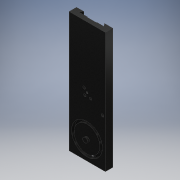
# Autodesk Inventor part: slide ontop of saddle
Saved by Autodesk Inventor 2018 (Build 220112000, 112)
## iProperties
Created: 2017-05-09
Part Number: slide ontop of saddle
Material: Steel, Cast
Document SubType Name: Modeling
Designer: m227586
Density: 7.85 g/cm^3
Appearance: Black Cast
Author: m227586
Autodesk Inventor part; units mm, degrees
ref_plane "YZ Plane" through (0, 0, 0) normal (1, 0, 0) x (0, 1, 0)
ref_plane "XZ Plane" through (0, 0, 0) normal (0, 1, 0) x (-1, 0, 0)
ref_plane "XY Plane" through (0, 0, 0) normal (0, 0, 1) x (1, 0, 0)
sketch "Sketch1" plane through (0, 0, 0) normal (0, 0, 1) x (1, 0, 0)
  line L0 (-7.7614, 0) -> (138.2386, 0)
  line L1 (138.2386, 0) -> (138.2386, 29.6)
  line L2 (-7.7614, 29.6) -> (-7.7614, 0)
  line L3 (-7.7614, 29.6) -> (22.1386, 29.6)
  line L4 (12.489, 18.1) -> (114.8883, 18.1)
  line L5 (22.1386, 29.6) -> (12.489, 18.1)
  line L6 (22.1386, 29.6) -> (41.4586, 29.6) construction
  line L7 (138.2386, 29.6) -> (105.2386, 29.6)
  line L8 (105.2386, 29.6) -> (114.8883, 18.1)
  point P0 (0, 0)
  dimension "d0" = 146
  dimension "d1" = 29.6
  dimension "d2" = 29.9
  dimension "d4" = 130
  dimension "d5" = 33
  dimension "d6" = 50
  constraints: 18 end point, 4 horizontal, 2 perpendicular
  measures "d0" distance of L0.start L0.end
  measures "d1" distance of L0.end L1.end
  measures "d2" distance of L2.start L3.end
  measures "d4" angle of L5 L6
  measures "d5" distance of L1.end L7.end
  measures "d6" angle of L8 L7
extrude "Extrusion1" add sketch "Sketch1" against normal blind 486
sketch "Sketch2" plane through (-7.7614, 29.6, 0) normal (0, 1, 0) x (1, 0, 0)
  line L0 (113, 0) -> (122.6496, 0) projected
  line L1 (124, 486) -> (113, 0)
  line L2 (113, 0) -> (113, 486) projected
  line L3 (113, 486) -> (124, 486)
  line L4 (122.6496, 0) -> (122.6496, 486) projected
  line L5 (113, 486) -> (113, 0)
  line L6 (146, 0) -> (146, 486) projected
  point P0 (7.7614, 0)
  dimension "d9" = 22
  constraints: 6 end point, 1 parallel, 1 perpendicular
  measures "d9" distance of L6.end L1.start
sketch "Sketch3" plane through (-7.7614, 0, 0) normal (0, -1, 0) x (1, 0, 0)
  line L0 (20.2504, -486) -> (122.6496, -486) projected
  line L1 (0, 0) -> (146, 0) projected
  circle A0 centre (71.6943, -409.4001) radius 62.1
  line L2 (71.45, -486) -> (71.4962, -471.5001)
  circle A1 centre (71.6943, -409.4001) radius 52
  circle A2 centre (71.6943, -409.4001) radius 9.51
  circle A3 centre (72.1613, -247.2004) radius 4.1
  point P0 (7.7614, 0)
  dimension "d10" = 124.2
  dimension "d11" = 14.5
  dimension "d12" = 62.1
  dimension "d13" = 104
  dimension "d14" = 19.02
  dimension "d15" = 8.2
  constraints: 4 centre point, 2 coincident, 2 end point, 1 midpoint
  measures "d10" diameter of A0
  measures "d11" distance of L2.start L2.end
  measures "d12" vertical distance of A0.centre L2.end
  measures "d13" diameter of A1
  measures "d14" diameter of A2
  measures "d15" diameter of A3
extrude "Extrusion2" cut sketch "Sketch3" against normal blind 13 contours A0
extrude "Extrusion3" add sketch "Sketch3" along normal blind 7.5 contours A2
extrude "Extrusion4" cut sketch "Sketch3" against normal through all contours A3
sketch "Sketch4" plane through (12.489, 18.1, 0) normal (0, 1, 0) x (1, 0, 0)
  circle A0 centre (51.911, 247.2004) radius 4.1 projected
  circle A1 centre (51.911, 247.2004) radius 9.5
  line L0 (0, 486) -> (102.3993, 486) projected
  line L1 (51.1996, 486) -> (51.1996, 476.6)
  arc A2 (46.6496, 476.6) -> (46.6496, 457.9) centre (46.6496, 467.25) ccw
  arc A3 (55.7496, 457.9) -> (55.7496, 476.6) centre (55.7496, 467.25) ccw
  line L2 (46.6496, 476.6) -> (55.7496, 476.6)
  line L3 (46.6496, 457.9) -> (55.7496, 457.9)
  circle A4 centre (51.1996, 411.4) radius 8.5
  point P0 (-12.489, 0)
  point P1 (51.1996, 476.6)
  dimension "d23" = 19
  dimension "d26" = 9.4
  dimension "d29" = 0
  dimension "d30" = 18.7
  dimension "d31" = 18.7
  dimension "d38" = 17
  dimension "d39" = 46.5
  constraints: 6 end point, 4 centre point, 4 point on circle, 2 coincident, 1 horizontal, 1 midpoint, 1 parallel, 1 vertical
  measures "d23" diameter of A1
  measures "d26" distance of L1.start L1.end
  measures "d29" distance from line of point (51.2, 476.6) L1
  measures "d30" diameter of A2
  measures "d31" diameter of A3
  measures "d38" diameter of A4
  measures "d39" distance from line of A4.centre L3
extrude "Extrusion5" cut sketch "Sketch4" against normal blind 3.7 contours A1
extrude "Extrusion7" cut sketch "Sketch4" against normal blind 6 contours L2 A3 L3 A2
extrude "Extrusion8" cut sketch "Sketch4" against normal blind 3 contours A4
sketch "Sketch5" plane through (-7.7614, 0, 0) normal (0, -1, 0) x (1, 0, 0)
  point P0 (7.7614, 0)
sketch "Sketch6" plane through (-7.7614, 0, 0) normal (0, -1, 0) x (1, 0, 0)
  circle A0 centre (86, -261) radius 5
  line L0 (146, -486) -> (0, -486) projected
  line L1 (146, 0) -> (146, -486) projected
  circle A1 centre (60.5, -235.5) radius 5.5
  line L2 (0, 0) -> (0, -486) projected
  circle A2 centre (134.5, -295.5) radius 5.5
  point P0 (7.7614, 0)
  dimension "d42" = 10
  dimension "d43" = 225
  dimension "d44" = 60
  dimension "d45" = 11
  dimension "d46" = 60.5
  dimension "d47" = 250.5
  dimension "d48" = 11
  dimension "d49" = 190.5
  dimension "d50" = 11.5
  constraints: 3 centre point, 3 coincident
  measures "d42" diameter of A0
  measures "d43" distance from line of L0 A0.centre
  measures "d44" distance from line of L1 A0.centre
  measures "d45" diameter of A1
  measures "d46" distance from line of L2 A1.centre
  measures "d47" distance from line of L0 A1.centre
  measures "d48" diameter of A2
  measures "d49" distance from line of L0 A2.centre
  measures "d50" distance from line of L1 A2.centre
hole "Hole1" at (126.7386, 0, -295.5) direction (0, 1, 0) diameter 8.5 end through all counterbore diameter 11 counterbore depth 8.5
hole "Hole2" at (78.2386, 0, -261) direction (0, 1, 0) diameter 7 end through all counterbore diameter 10 counterbore depth 7.5
hole "Hole3" at (52.7386, 0, -235.5) direction (0, 1, 0) diameter 7.5 end through all counterbore diameter 11 counterbore depth 7
thread "Thread1" size "M9x1.25" class "6H" standard "ANSI Metric M Profile" full length
sketch "Sketch14" plane through (12.489, 18.1, 0) normal (0, 1, 0) x (1, 0, 0)
  circle A0 centre (51.911, 247.2004) radius 4.1 construction
  line L0 (51.911, 247.2004) -> (92.7496, 247.2004) construction
  line L1 (92.7496, 0) -> (92.7496, 486) construction
  line L2 (92.7496, 247.2004) -> (92.7496, 208.2004) construction
  line L3 (92.7496, 208.2004) -> (9.6496, 208.2004)
  line L4 (9.6496, 208.2004) -> (9.6496, 272.2004)
  line L5 (9.6496, 272.2004) -> (92.7496, 272.2004)
  line L6 (92.7496, 272.2004) -> (92.7496, 208.2004)
  point P0 (-12.489, 0)
  dimension "d82" = 39
  dimension "d83" = 83.1
  dimension "d84" = 64
  constraints: 12 end point, 2 horizontal, 2 parallel, 2 perpendicular, 1 point on line
  measures "d82" distance of L0.end L2.end
  measures "d83" distance of L4.end L5.end
  measures "d84" distance of L3.end L4.end
extrude "Extrusion11" cut sketch "Sketch14" against normal blind 6
sketch "Sketch15" plane through (12.489, 12.1, 0) normal (0, 1, 0) x (1, 0, 0)
  circle A0 centre (65.7496, 261) radius 3.5 projected
  point P0 (-12.489, 0)
  point P1 (43.0496, 261)
  dimension "d87" = 22.7
  measures "d87" distance of A0.centre point (43.05, 261)
hole "Hole4" at (55.5386, 12.1, -261) direction (0, -1, 0) diameter 7 end through all
sketch "Sketch16" plane through (-7.7614, 0, 0) normal (0, -1, 0) x (1, 0, 0)
  circle A0 centre (63.3, -261) radius 3.5 projected
  circle A1 centre (63.3, -261) radius 5
  point P0 (7.7614, 0)
  dimension "d95" = 10
  constraints: 1 centre point, 1 coincident
  measures "d95" diameter of A1
extrude "Extrusion12" cut sketch "Sketch16" against normal blind 7.5
sketch "Sketch17" plane through (12.489, 18.1, 0) normal (0, 1, 0) x (1, 0, 0)
  line L0 (92.7496, 0) -> (92.7496, 486) construction
  line L1 (92.7496, 0) -> (73.3996, 0) construction
  line L2 (-20.2504, 0) -> (125.7496, 0) construction
  line L3 (73.3996, 0) -> (35.3996, 0)
  line L4 (35.3996, 0) -> (35.3996, 145)
  line L5 (35.3996, 145) -> (73.3996, 145)
  line L6 (73.3996, 145) -> (73.3996, 0)
  point P0 (-12.489, 0)
  dimension "d99" = 19.35
  dimension "d100" = 38
  dimension "d101" = 145
  constraints: 10 end point, 2 parallel, 1 horizontal, 1 perpendicular, 1 point on line
  measures "d99" distance of L0.start L1.end
  measures "d100" distance of L4.end L5.end
  measures "d101" distance of L3.end L4.end
extrude "Extrusion13" cut sketch "Sketch17" against normal blind 2
body "Solid1"
